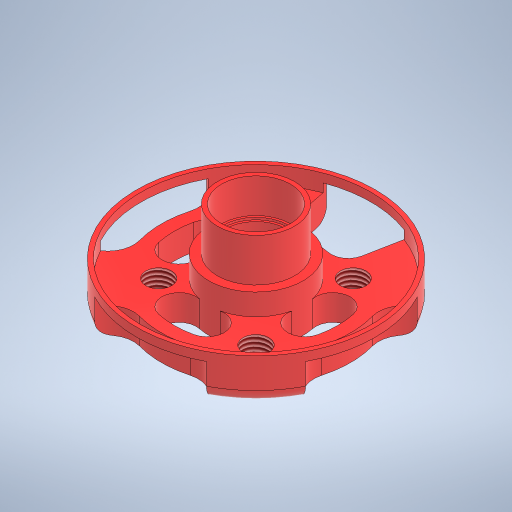
# Autodesk Inventor part: BASE
Saved by Autodesk Inventor 2023.4 (Build 274418000, 418)
## iProperties
Created: 2024-01-31
Part Number: BASE
Material: Aluminum 6061
Document SubType Name: Modeling
Designer: Nathan Cai
Density: 2.7 g/cm^3
Appearance: Light Red
Author: Nathan Cai
Autodesk Inventor part; units mm, degrees
ref_plane "YZ Plane" through (0, 0, 0) normal (1, 0, 0) x (0, 1, 0)
ref_plane "XZ Plane" through (0, 0, 0) normal (0, 1, 0) x (-1, 0, 0)
ref_plane "XY Plane" through (0, 0, 0) normal (0, 0, 1) x (1, 0, 0)
sketch "Sketch1" plane through (0, 0, 0) normal (1, 0, 0) x (0, 1, 0)
  line L0 (0, 0) -> (10.5, 0)
  line L1 (10.5, 0) -> (10.5, -4)
  line L2 (10.5, -4) -> (0, -4)
  line L3 (0, -4) -> (0, 0)
  line L4 (0, -4) -> (10.5, -4)
  line L5 (10.5, -4) -> (10.5, -4.5)
  line L6 (10.5, -4.5) -> (0, -4.5)
  line L7 (0, -4.5) -> (0, -4)
  line L8 (0, -4.5) -> (5.5, -4.5)
  line L9 (5.5, -4.5) -> (5.5, -5.5)
  line L10 (5.5, -5.5) -> (0, -5.5)
  line L11 (0, -5.5) -> (0, -4.5)
  line L12 (0, -5.5) -> (3, -5.5)
  line L13 (3, -5.5) -> (3, -13.875)
  line L14 (3, -13.875) -> (0, -13.875)
  line L15 (0, -13.875) -> (0, -5.5)
  line L16 (3, -13.875) -> (5, -13.875)
  line L17 (5, -13.875) -> (5, -13.375)
  line L18 (5, -13.375) -> (3, -13.375)
  line L19 (3, -13.375) -> (3, -13.875)
  line L20 (6.25, -4) -> (4.25, -4)
  line L21 (4.25, -4) -> (4.25, -3.5)
  line L22 (4.25, -3.5) -> (6.25, -3.5)
  line L23 (6.25, -3.5) -> (6.25, -4)
  line L24 (6.25, -4) -> (6.5, -4)
  line L25 (6.5, -4) -> (6.5, -3.75)
  line L26 (6.5, -3.75) -> (6.25, -3.75)
  line L27 (6.25, -3.75) -> (6.25, -4)
  line L28 (4.25, -4) -> (4, -4)
  line L29 (4, -4) -> (4, -3.75)
  line L30 (4, -3.75) -> (4.25, -3.75)
  line L31 (4.25, -3.75) -> (4.25, -4)
  dimension "d0" = 10.5
  dimension "d1" = 4
  dimension "d2" = 0.5
  dimension "d3" = 5.5
  dimension "d4" = 5.5
  dimension "d5" = 3
  dimension "d6" = 13.875
  dimension "d7" = 2
  dimension "d8" = 0.5
  dimension "d48" = 3.5
  dimension "d49" = 4.25
  dimension "d50" = 4.25
  dimension "d51" = 0.25
  dimension "d52" = 0.25
  dimension "d53" = 0.25
  dimension "d54" = 0.25
  constraints: 64 end point, 16 parallel, 8 horizontal, 8 perpendicular, 2 point on line
  measures "d0" distance of L1.end L2.end
  measures "d1" distance of L0.end L1.end
  measures "d2" distance of L4.end L5.end
  measures "d3" distance of L9.end L10.end
  measures "d4" distance between parallel lines of L0 L10
  measures "d5" distance of L13.end L14.end
  measures "d6" distance between parallel lines of L0 L14
  measures "d7" distance of L18.end L17.end
  measures "d8" distance of L17.end L16.end
  measures "d48" distance between parallel lines of L0 L22
  measures "d49" distance between parallel lines of L3 L21
  measures "d50" distance between parallel lines of L1 L23
  measures "d51" distance of L26.end L25.end
  measures "d52" distance of L25.end L24.end
  measures "d53" distance of L29.end L30.end
  measures "d54" distance of L28.end L29.end
revolve "Revolution1" add sketch "Sketch1" angle 360 about axis through (0, 0, 0) along (0, 1, 0) contours L2 L5 L6 L7 | L29 L30 L21 L2 | L6 L9 L10 L11 | L2 L23 L26 L25 | L21 L22 L23 L2 | L10 L13 L14 L15 | L18 L17 L16 L13
fillet "Fillet1" radius 1.5 1 edges at (0, 0, 13.875)
sketch "Sketch2" plane through (0, 0, 0) normal (0, -1, 0) x (1, 0, 0)
  circle A0 centre (0, 0) radius 5.5 construction
  line L0 (0, 0) -> (0, -5.5) construction
  circle A1 centre (0, 0) radius 5.5 projected
  line L1 (0, 0) -> (-8.7504, -8.7504) construction
  circle A2 centre (0, 0) radius 12.375 construction
  circle A3 centre (0, 0) radius 8 construction
  circle A4 centre (0, 0) radius 9.5 construction
  circle A5 centre (-6.7175, -6.7175) radius 1.5
  line L2 (0, 0) -> (-5.6569, 5.6569) construction
  circle A6 centre (-5.6569, 5.6569) radius 1.5
  circle A7 centre (5.6569, -5.6569) radius 1.5
  circle A8 centre (6.7175, 6.7175) radius 1.5
  arc A9 (1.6233, 7.3222) -> (-1.6233, 7.3222) centre (0, 0) ccw construction
  arc A10 (2.0562, 9.2748) -> (-2.0562, 9.2748) centre (0, 0) ccw
  arc A11 (1.1904, 5.3696) -> (-1.1904, 5.3696) centre (0, 0) ccw
  arc A12 (1.1904, 5.3696) -> (2.0562, 9.2748) centre (1.6233, 7.3222) ccw
  arc A13 (-2.0562, 9.2748) -> (-1.1904, 5.3696) centre (-1.6233, 7.3222) ccw
  line L3 (-1.6233, 7.3222) -> (0, 0) construction
  line L4 (0, 0) -> (0, 7.5) construction
  line L5 (1.6233, 7.3222) -> (0, 0) construction
  arc A14 (-5.3696, 1.1904) -> (-9.2748, 2.0562) centre (-7.3222, 1.6233) ccw
  arc A15 (-7.3222, 1.6233) -> (-7.3222, -1.6233) centre (0, 0) ccw construction
  arc A16 (-9.2748, 2.0562) -> (-9.2748, -2.0562) centre (0, 0) ccw
  arc A17 (-9.2748, -2.0562) -> (-5.3696, -1.1904) centre (-7.3222, -1.6233) ccw
  arc A18 (-5.3696, 1.1904) -> (-5.3696, -1.1904) centre (0, 0) ccw
  arc A19 (-1.1904, -5.3696) -> (-2.0562, -9.2748) centre (-1.6233, -7.3222) ccw
  arc A20 (-1.6233, -7.3222) -> (1.6233, -7.3222) centre (0, 0) ccw construction
  arc A21 (-2.0562, -9.2748) -> (2.0562, -9.2748) centre (0, 0) ccw
  arc A22 (2.0562, -9.2748) -> (1.1904, -5.3696) centre (1.6233, -7.3222) ccw
  arc A23 (-1.1904, -5.3696) -> (1.1904, -5.3696) centre (0, 0) ccw
  arc A24 (5.3696, -1.1904) -> (9.2748, -2.0562) centre (7.3222, -1.6233) ccw
  arc A25 (7.3222, -1.6233) -> (7.3222, 1.6233) centre (0, 0) ccw construction
  arc A26 (9.2748, -2.0562) -> (9.2748, 2.0562) centre (0, 0) ccw
  arc A27 (9.2748, 2.0562) -> (5.3696, 1.1904) centre (7.3222, 1.6233) ccw
  arc A28 (5.3696, -1.1904) -> (5.3696, 1.1904) centre (0, 0) ccw
  arc A29 (3.7631, 13.4848) -> (-3.7631, 13.4848) centre (0, 0) ccw construction
  arc A30 (4.5695, 16.3744) -> (-4.5695, 16.3744) centre (0, 0) ccw
  arc A31 (2.9567, 10.5952) -> (-2.9567, 10.5952) centre (0, 0) ccw
  arc A32 (2.9567, 10.5952) -> (4.5695, 16.3744) centre (3.7631, 13.4848) ccw
  arc A33 (-4.5695, 16.3744) -> (-2.9567, 10.5952) centre (-3.7631, 13.4848) ccw
  line L6 (0, 0) -> (6.4128, 12.0779) construction
  arc A34 (10.5952, -2.9567) -> (10.5952, 2.9567) centre (0, 0) ccw
  arc A35 (16.3744, 4.5695) -> (10.5952, 2.9567) centre (13.4848, 3.7631) ccw
  arc A36 (10.5952, -2.9567) -> (16.3744, -4.5695) centre (13.4848, -3.7631) ccw
  arc A37 (16.3744, -4.5695) -> (16.3744, 4.5695) centre (0, 0) ccw
  arc A38 (13.4848, -3.7631) -> (13.4848, 3.7631) centre (0, 0) ccw construction
  arc A39 (-2.9567, -10.5952) -> (2.9567, -10.5952) centre (0, 0) ccw
  arc A40 (4.5695, -16.3744) -> (2.9567, -10.5952) centre (3.7631, -13.4848) ccw
  arc A41 (-2.9567, -10.5952) -> (-4.5695, -16.3744) centre (-3.7631, -13.4848) ccw
  arc A42 (-4.5695, -16.3744) -> (4.5695, -16.3744) centre (0, 0) ccw
  arc A43 (-3.7631, -13.4848) -> (3.7631, -13.4848) centre (0, 0) ccw construction
  arc A44 (-10.5952, 2.9567) -> (-10.5952, -2.9567) centre (0, 0) ccw
  arc A45 (-16.3744, -4.5695) -> (-10.5952, -2.9567) centre (-13.4848, -3.7631) ccw
  arc A46 (-10.5952, 2.9567) -> (-16.3744, 4.5695) centre (-13.4848, 3.7631) ccw
  arc A47 (-16.3744, 4.5695) -> (-16.3744, -4.5695) centre (0, 0) ccw
  arc A48 (-13.4848, 3.7631) -> (-13.4848, -3.7631) centre (0, 0) ccw construction
  circle A49 centre (0, 0) radius 2.25 construction
  arc A50 (-1.948, -8.7867) -> (1.948, -8.7867) centre (0, 0) ccw construction
  arc A51 (-2.3808, -10.7393) -> (2.3808, -10.7393) centre (0, 0) ccw
  arc A52 (-1.5151, -6.8341) -> (1.5151, -6.8341) centre (0, 0) ccw
  arc A53 (-1.5151, -6.8341) -> (-2.3808, -10.7393) centre (-1.948, -8.7867) ccw
  arc A54 (2.3808, -10.7393) -> (1.5151, -6.8341) centre (1.948, -8.7867) ccw
  line L7 (2.2093, 0.4258) -> (5.3775, -16.0134)
  line L8 (-2.2093, 0.4258) -> (-5.3775, -16.0134)
  point P0 (-7.5, 0)
  point P1 (0, -7.5)
  point P2 (7.5, 0)
  point P3 (12.0779, -6.4128)
  point P4 (-6.4128, -12.0779)
  point P5 (-12.0779, 6.4128)
  point P6 (5.3696, 1.1904)
  point P7 (1.1904, 5.3696)
  point P8 (-1.1904, 5.3696)
  point P9 (-5.3696, 1.1904)
  point P10 (-5.3696, -1.1904)
  point P11 (-1.1904, -5.3696)
  point P12 (1.1904, -5.3696)
  point P13 (5.3696, -1.1904)
  point P14 (5.2926, -16.0656)
  point P15 (2.2117, 0.4135)
  point P16 (-2.2117, 0.4135)
  point P17 (4.5121, -11.5231)
  point P18 (-4.5121, -11.5231)
  point P19 (3.9118, -8.4082)
  point P20 (-3.9118, -8.4082)
  dimension "d11" = 11
  dimension "d13" = 16
  dimension "d14" = 19
  dimension "d12" = 45
  dimension "d15" = 3
  dimension "d16" = 3
  dimension "d19" = 360
  dimension "d21" = 4
  dimension "d24" = 25
  dimension "d27" = 360
  dimension "d29" = 11
  dimension "d30" = 3
  dimension "d33" = 360
  dimension "d37" = 4.5
  dimension "d38" = 4
  dimension "d39" = 7
  constraints: 105 point on circle, 50 centre point, 18 end point, 16 tangent, 10 coincident, 5 point on line, 3 symmetric about line, 2 vertical, 1 perpendicular, 130 other
  measures "d12" angle of L0 L1
  measures "d15" diameter of A5
  measures "d16" diameter of A6
  measures "d24" angle of L5 L3
  measures "d29" radius of A31
  measures "d30" radius of A33
  measures "d37" diameter of A49
  measures "d38" diameter of A53
  measures "d39" radius of A52
extrude "Extrusion1" cut sketch "Sketch2" against normal blind 4 contours A1 A27 A26 A24 | A1 A13 A10 A12 | L7 A40 A39 A54 | A54 A39 A53 A19 A21 A22 | A1 A17 A16 A14 | A22 A21 A19 A53 A52 A54 | A39 A40 L7 A42 A41 L8 | A39 A41 L8 A53 | A5 | A6 | A7 | A8 | A32 A31 A33 A30 | A34 A35 A37 A36 | A44 A45 A47 A46
thread "Thread1" size "M3x0.5" class "6H" standard "ANSI Metric M Profile" length 3
thread "Thread2" size "M3x0.5" class "6H" standard "ANSI Metric M Profile" length 5.0038
thread "Thread3" size "M3x0.5" class "6H" standard "ANSI Metric M Profile" length 5.0038
thread "Thread4" size "M3x0.5" class "6H" standard "ANSI Metric M Profile" length 5.0038
equation "\"d49\" = d50"
body "Solid1"
